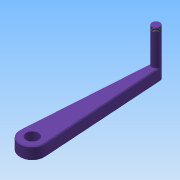
# Autodesk Inventor part: 刀轴带动盘连杆
Saved by Autodesk Inventor 2015 (Build 190159000, 159)
## iProperties
Created: 2017-05-26
Part Number: 刀轴带动盘连杆
Material: 常规
Document SubType Name: Modeling
Designer: Administrator
Density: 1 g/cm^3
Appearance: 紫罗兰色
Author: Administrator
Autodesk Inventor part; units mm, degrees
ref_plane "YZ Plane" through (0, 0, 0) normal (1, 0, 0) x (0, 1, 0)
ref_plane "XZ Plane" through (0, 0, 0) normal (0, 1, 0) x (-1, 0, 0)
ref_plane "XY Plane" through (0, 0, 0) normal (0, 0, 1) x (1, 0, 0)
sketch "草图1" plane through (0, 0, 0) normal (0, 0, 1) x (1, 0, 0)
  circle A0 centre (0, 0) radius 15
  circle A1 centre (0, 150) radius 5
  line L0 (0, 150) -> (0, 0)
  line L1 (-14.96663, 1) -> (-4.988877, 150.333333)
  line L2 (4.988877, 150.333333) -> (14.96663, 1)
  dimension "d0" = 30
  dimension "d1" = 10
  dimension "d2" = 150
  constraints: 6 end point, 4 point on circle, 4 tangent, 2 centre point, 1 coincident, 1 vertical
  measures "d0" diameter of A0
  measures "d1" diameter of A1
  measures "d2" distance of L0.start L0.end
extrude "拉伸1" add sketch "草图1" along normal blind 15
sketch "草图2" plane through (0, 0, 15) normal (0, 0, 1) x (1, 0, 0)
  circle A0 centre (0, 0) radius 7.5
  dimension "d5" = 15
  constraints: 1 centre point, 1 coincident
  measures "d5" diameter of A0
extrude "拉伸2" cut sketch "草图2" against normal through all
sketch "草图3" plane through (0, 0, 15) normal (0, 0, 1) x (1, 0, 0)
  circle A0 centre (0, 150) radius 5
  arc A1 (4.988877, 150.333333) -> (-4.988877, 150.333333) centre (0, 150) ccw
  point P0 (0, 0)
  dimension "d8" = 10
  constraints: 1 centre point, 1 concentric
  measures "d8" diameter of A0
extrude "拉伸3" add sketch "草图3" along normal blind 42.5
thread "螺纹1" size "M10x1.5" class "6g" standard "ANSI Metric M Profile" length 5
chamfer "倒角1" distance 0.25 angle 45 1 edges at (-5, 150, 57.5)
chamfer "倒角2" distance 1 angle 45 7 edges at (9.9778, 75.6667, 15) (0, -15, 15) (-9.9778, 75.6667, 15) (9.9778, 75.6667, 0) (0, 155, 0) (-9.9778, 75.6667, 0) (0, -15, 0)
chamfer "倒角3" distance 0.25 angle 45 1 edges at (-5, 150, 57.25)
equation "\"d6\" = d5"
